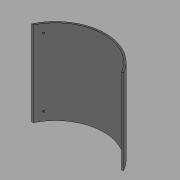
# Autodesk Inventor part: security_cover
Saved by Autodesk Inventor 2019 (Build 230136000, 136)
## iProperties
Part Number: security_cover
Material: Generic
Document SubType Name: Modeling
Designer: Javi
Appearance: Default
Author: Javi
Autodesk Inventor part; units mm, degrees
ref_plane "XZ Plane" through (0, 0, 0) normal (0, 1, 0) x (-1, 0, 0)
ref_plane "XY Plane" through (0, 0, 0) normal (0, 0, 1) x (1, 0, 0)
sketch "Sketch2" plane through (0, 0, 0) normal (0, 1, 0) x (-1, 0, 0)
  arc A0 (-102.191, -59) -> (106.8951, -49.9743) centre (0, 0) ccw
  arc A1 (-98.7269, -57) -> (102.4625, -49.9743) centre (0, 0) ccw
  line L0 (-98.7269, -57) -> (-102.191, -59)
  line L1 (102.4625, -49.9743) -> (106.8951, -49.9743)
  line L2 (102.4625, -49.9743) -> (106.0577, -51.7278)
  dimension "d9" = 4
  dimension "d10" = 118
  dimension "d14" = 150
  dimension "d15" = 26
  constraints: 6 end point, 5 point on circle, 4 line through centre, 2 centre point, 1 coincident, 1 horizontal
  measures "d9" radial gap between concentric circles of A0 A1
  measures "d10" radius of A0
  measures "d14" angle of L1 L0
  measures "d15" angle of L1 L2
extrude "Extrusion1" add sketch "Sketch2" along normal blind 200
ref_plane "Work Plane1" through (-118, 0, 0) normal (1, 0, 0) x (0, 1, 0)
sketch "Sketch3" plane through (-118, 0, 0) normal (1, 0, 0) x (0, 1, 0)
  circle A0 centre (180, -55.9743) radius 2
  line L0 (0, -49.9743) -> (200, -49.9743) projected
  line L1 (200, -118) -> (200, -49.9743) projected
  circle A1 centre (20, -55.9743) radius 2
  point P0 (0, 0)
  point P1 (200, -59)
  dimension "d16" = 4
  dimension "d17" = 6
  dimension "d21" = 160
  dimension "d43" = 20
  constraints: 2 centre point, 1 horizontal, 2 other
  measures "d16" diameter of A0
  measures "d17" distance from line of L0 A0.centre
  measures "d21" distance of A0.centre A1.centre
  measures "d43" distance from line of L1 A0.centre
sketch "Sketch4" plane through (-118, 0, 0) normal (1, 0, 0) x (0, 1, 0)
  line L0 (23.5, -52.4743) -> (16.5, -52.4743)
  line L1 (16.5, -52.4743) -> (16.5, -59.4743)
  line L2 (16.5, -59.4743) -> (23.5, -59.4743)
  line L3 (23.5, -59.4743) -> (23.5, -52.4743)
  line L4 (0, -49.9743) -> (200, -49.9743) projected
  line L5 (0, -118) -> (0, -49.9743) projected
  line L6 (183.5, -52.4743) -> (176.5, -52.4743)
  line L7 (176.5, -52.4743) -> (176.5, -59.4743)
  line L8 (176.5, -59.4743) -> (183.5, -59.4743)
  line L9 (183.5, -59.4743) -> (183.5, -52.4743)
  point P0 (0, 0)
  point P1 (0, -59)
  dimension "d28" = 7
  dimension "d29" = 7
  dimension "d34" = 160
  dimension "d39" = 2.5
  dimension "d40" = 16.5
  constraints: 16 end point, 2 horizontal, 2 parallel, 1 perpendicular, 9 other
  measures "d28" distance of L2.end L1.end
  measures "d29" distance of L1.end L0.end
  measures "d34" distance of L0.start L6.start
  measures "d39" distance between parallel lines of L4 L0
  measures "d40" distance between parallel lines of L5 L1
derived "inner_mechanism.ipt"
ref_plane "Work Plane8" through (-102.4625, 0, -49.9743) normal (-0.8350088, 0, -0.5502366) x (0, 1, 0)
sketch "Sketch9" plane through (-102.4625, 0, -49.9743) normal (-0.8350088, 0, -0.5502366) x (0, 1, 0)
  circle A0 centre (20, 18) radius 2
  line L0 (0, 0) -> (200, 0) projected
  line L1 (0, 128.6496) -> (0, 0) projected
  circle A1 centre (180, 18) radius 2
  point P0 (0, 14.6496)
  point P1 (0, 116.5683)
  dimension "d88" = 4
  dimension "d89" = 18
  dimension "d90" = 20
  dimension "d93" = 160
  constraints: 2 centre point, 1 horizontal, 2 other
  measures "d88" diameter of A0
  measures "d89" distance from line of L0 A0.centre
  measures "d90" distance from line of L1 A0.centre
  measures "d93" distance of A0.centre A1.centre
extrude "Extrusion8" cut sketch "Sketch9" along normal through all both and the other way through all
ref_plane "Work Plane9" through (-98.531, 0, -64.9279) normal (-0.8350088, 0, -0.5502366) x (0, -1, 0)
sketch "Sketch10" plane through (-98.531, 0, -64.9279) normal (-0.8350088, 0, -0.5502366) x (0, -1, 0)
  line L0 (-22, -5.4114) -> (-18, -5.4114)
  line L1 (-18, -5.4114) -> (-18, -1.4114)
  line L2 (-18, -1.4114) -> (-22, -1.4114)
  line L3 (-22, -1.4114) -> (-22, -5.4114)
  line L4 (0, 17.0886) -> (-200, 17.0886) projected
  line L5 (0, 17.0886) -> (0, -118) projected
  line L6 (-182, -5.4114) -> (-178, -5.4114)
  line L7 (-178, -5.4114) -> (-178, -1.4114)
  line L8 (-178, -1.4114) -> (-182, -1.4114)
  line L9 (-182, -1.4114) -> (-182, -5.4114)
  point P0 (0, 0)
  point P1 (0, -105.4947)
  dimension "d100" = 4
  dimension "d101" = 4
  dimension "d102" = 18.5
  dimension "d103" = 18
  dimension "d106" = 160
  constraints: 16 end point, 2 horizontal, 2 parallel, 1 perpendicular, 8 other
  measures "d100" distance of L2.end L1.end
  measures "d101" distance of L1.end L0.end
  measures "d102" distance between parallel lines of L4 L2
  measures "d103" distance between parallel lines of L5 L1
  measures "d106" distance of L0.start L6.start
extrude "Extrusion9" cut sketch "Sketch10" against normal blind 0.5
ref_plane "Work Plane6" through (-62.727, 0, 95.191) normal (0.5502366, 0, -0.8350088) x (0, 1, 0)
body "Solid1"
